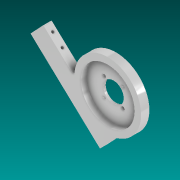
# Autodesk Inventor part: base frame voorkant 10 mm
Saved by Autodesk Inventor 2020.3 (Build 243373000, 373)
## iProperties
Created: 2020-05-20
Part Number: base frame voorkant 10 mm
Material: Aluminum 6061
Document SubType Name: Modeling
Designer: Svend
Density: 2.7 g/cm^3
Appearance: Aluminum - Polished
Author: Svend
Autodesk Inventor part; units mm, degrees
ref_plane "YZ Plane" through (0, 0, 0) normal (1, 0, 0) x (0, 1, 0)
ref_plane "XZ Plane" through (0, 0, 0) normal (0, 1, 0) x (-1, 0, 0)
ref_plane "Work Plane1" through (0, 0, 0) normal (0, 0, 1) x (1, 0, 0)
sketch "Sketch1" plane through (0, 0, 0) normal (0, 0, 1) x (1, 0, 0)
  arc A0 (-77.068, 33.987) -> (-78.4814, 33.9394) centre (-77.7509, 33.2565) ccw projected
  line L0 (-78.4814, 33.9394) -> (-92.9244, 18.4887) projected
  line L1 (-92.9244, 18.4887) -> (-9.2531, -59.7257) projected
  line L2 (-9.2531, -59.7257) -> (9.7389, -39.4086) projected
  arc A1 (10.6702, -38.8458) -> (9.7389, -39.4086) centre (11.2, -40.7744) ccw projected
  arc A2 (10.6702, -38.8458) -> (-40.1013, 3.8394) centre (0, 0) ccw projected
  line L3 (-43.4579, 2.5689) -> (-77.068, 33.987) projected
  circle A3 centre (33.3141, 1.123) radius 2.5 projected
  circle A4 centre (1.123, -33.3141) radius 2.5 projected
  circle A5 centre (0, 0) radius 21 projected
  circle A6 centre (-1.123, 33.3141) radius 2.5 projected
  circle A7 centre (-33.3141, -1.123) radius 2.5 projected
  circle A8 centre (0, 0) radius 12.5 projected
  circle A9 centre (0, -16) radius 2 projected
  circle A10 centre (0, 16) radius 2 projected
  circle A11 centre (-16, 0) radius 2 projected
  circle A12 centre (16, 0) radius 2 projected
  circle A13 centre (11.3137, 11.3137) radius 1.6 projected
  circle A14 centre (-11.3137, -11.3137) radius 1.6 projected
  circle A15 centre (-11.3137, 11.3137) radius 1.6 projected
  circle A16 centre (11.3137, -11.3137) radius 1.6 projected
  circle A17 centre (0, 0) radius 20.7 projected
  circle A18 centre (0, 0) radius 40.2846
  line L4 (31.6375, -97.9493) -> (-99.8575, 24.9697) projected
  arc A19 (-43.4579, 2.5689) -> (-40.1013, 3.8394) centre (-42.0921, 4.03) ccw projected
  point P0 (0, 0)
  point P1 (-45.0314, -26.2807)
  point P2 (-23.1886, -46.699)
  point P3 (0, 0)
  point P4 (10.6702, -38.8458)
  point P5 (-40.1013, 3.8394)
  point P6 (0, 0)
  constraints: 1 centre point, 1 coincident
extrude "Extrusion1" add sketch "Sketch1" along normal blind 10 contours L3 A19 A18 A1 L2 L1 L0 A0 | A2 A18 | A3 | A4 | A5 | A6 | A7 | A9 | A10 | A11 | A12 | A13 | A14 | A15 | A16 | A17
sketch "Sketch2" plane through (-77.068, 33.987, 10) normal (0.6828833, 0.7305275, 0) x (0.7305275, -0.6828833, 0)
  arc A0 (36.818, 70.5) -> (34.818, 72.5) centre (34.818, 70.5) ccw projected
  line L0 (-3.182, 72.5) -> (34.818, 72.5) projected
  arc A1 (-3.182, 72.5) -> (-5.182, 70.5) centre (-3.182, 70.5) ccw projected
  line L1 (-5.182, 2) -> (-5.182, 70.5) projected
  arc A2 (-5.182, 2) -> (-3.182, 0) centre (-3.182, 2) ccw projected
  line L2 (34.818, 0) -> (-3.182, 0) projected
  arc A3 (34.818, 0) -> (36.818, 2) centre (34.818, 2) ccw projected
  line L3 (36.818, 70.5) -> (36.818, 2) projected
  circle A4 centre (15.818, 36.25) radius 12.6 projected
  circle A5 centre (31.818, 36.25) radius 2 projected
  arc A6 (31.218, 2.9) -> (31.218, 7.1) centre (31.218, 5) ccw projected
  line L4 (0.418, 2.9) -> (31.218, 2.9) projected
  arc A7 (0.418, 7.1) -> (0.418, 2.9) centre (0.418, 5) ccw projected
  line L5 (31.218, 7.1) -> (0.418, 7.1) projected
  circle A8 centre (15.818, 20.25) radius 2 projected
  arc A9 (0.418, 69.6) -> (0.418, 65.4) centre (0.418, 67.5) ccw projected
  line L6 (31.218, 69.6) -> (0.418, 69.6) projected
  arc A10 (31.218, 65.4) -> (31.218, 69.6) centre (31.218, 67.5) ccw projected
  line L7 (0.418, 65.4) -> (31.218, 65.4) projected
  circle A11 centre (15.818, 52.25) radius 2 projected
  circle A12 centre (-0.182, 36.25) radius 2 projected
  circle A13 centre (7.918, 67.5) radius 1.5706 projected
  circle A14 centre (23.718, 67.5) radius 1.5706 projected
  circle A15 centre (28.5459, 23.5221) radius 2 projected
  circle A16 centre (3.09, 23.5221) radius 2 projected
  circle A17 centre (3.09, 48.9779) radius 2 projected
  circle A18 centre (28.5459, 48.9779) radius 2 projected
  point P0 (79.5095, 10)
  point P1 (7.918, 5)
  point P2 (23.718, 5)
  constraints: 2 horizontal alignment, 2 vertical alignment
hole "Hole1" at (-71.2837, 28.58, 5) at (-59.7414, 17.7904, 5) direction (-0.6828833, -0.7305275, 0) diameter 3.242 end through all thread size "M4x0.7" class "6H" standard "ISO Metric profile"
sketch "Sketch9" plane through (0, 0, 10) normal (0, 0, 1) x (1, 0, 0)
  circle A0 centre (0, 0) radius 32.55
  dimension "d44" = 65.1
  constraints: 1 centre point, 1 coincident
  measures "d44" diameter of A0
extrude "Extrusion4" cut sketch "Sketch9" against normal blind 7.1
sketch "Sketch11" plane through (-9.2531, -59.7257, 0) normal (-0.6828833, -0.7305275, 0) x (0.7305275, -0.6828833, 0)
  circle A0 centre (-60.5521, 5) radius 2.25 projected
  circle A1 centre (-7.5, 5) radius 2.25 projected
  point P0 (-34.026, 0)
hole "Hole7" at (-53.488, -18.3757, 5) at (-14.732, -54.604, 5) direction (0.6828833, 0.7305275, 0) diameter 3.242 depth 12.8 tip angle 118 thread size "M4x0.7" class "6H" standard "ISO Metric profile"
sketch "Sketch12" plane through (0, 0, 2.9) normal (0, 0, 1) x (1, 0, 0)
  circle A0 centre (0, 0) radius 12.5 projected
  circle A1 centre (0, -18) radius 2 projected
  circle A2 centre (0, 18) radius 2 projected
  circle A3 centre (-18, 0) radius 2 projected
  circle A4 centre (18, 0) radius 2 projected
  circle A5 centre (11.3137, 11.3137) radius 1.6 projected
  circle A6 centre (-11.3137, -11.3137) radius 1.6 projected
  circle A7 centre (-11.3137, 11.3137) radius 1.6 projected
  circle A8 centre (11.3137, -11.3137) radius 1.6 projected
  circle A9 centre (0, 0) radius 20.7 projected
  point P0 (0, 0)
hole "Hole8" at (11.3137, 11.3137, 2.9) at (-11.3137, 11.3137, 2.9) at (-11.3137, -11.3137, 2.9) at (11.3137, -11.3137, 2.9) direction (0, 0, -1) diameter 4.2 depth 12.8 tip angle 118 clearance for "Countersunk Flat Head Screw ISO 2009/7046" size "M4" standard "ISO"
body "Solid1"
